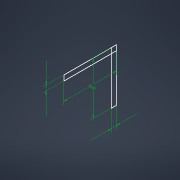
# Autodesk Inventor part: slide_panel_joint
Saved by Autodesk Inventor 2021 (Build 250183000, 183)
## iProperties
Created: 2023-03-31
Part Number: slide_panel_joint
Material: 一般
Document SubType Name: Modeling
Designer: casey
Density: 1 g/cm^3
Appearance: 既定
Author: casey
Autodesk Inventor part; units mm, degrees
ref_plane "YZ Plane" through (0, 0, 0) normal (1, 0, 0) x (0, 1, 0)
ref_plane "XZ Plane" through (0, 0, 0) normal (0, 1, 0) x (-1, 0, 0)
ref_plane "XY Plane" through (0, 0, 0) normal (0, 0, 1) x (1, 0, 0)
sketch "スケッチ1" plane through (0, 0, 0) normal (1, 0, 0) x (0, 1, 0)
  line L0 (0, 0) -> (-1, 0)
  line L1 (-1, 0) -> (-1, 10)
  line L2 (-1, 10) -> (0, 10)
  line L3 (0, 10) -> (0, 0)
  line L4 (0, 0) -> (-10, 0)
  line L5 (-10, 0) -> (-10, 1)
  line L6 (-10, 1) -> (0, 1)
  line L7 (0, 1) -> (0, 0)
  point P0 (-1, 1)
  dimension "d0" = 1
  dimension "d1" = 10
  dimension "d2" = 10
  dimension "d3" = 1
  constraints: 16 end point, 4 parallel, 2 horizontal, 2 perpendicular
  measures "d0" distance of L1.end L2.end
  measures "d1" distance of L0.end L1.end
  measures "d2" distance of L5.end L6.end
  measures "d3" distance of L4.end L5.end
extrude "押し出し1" add sketch "スケッチ1" along normal blind 130
sketch "スケッチ2" plane through (0, 0, 10) normal (0, 1, 0) x (1, 0, 0)
  line L0 (0, 10) -> (0, 0) projected
  line L1 (0, 10) -> (130, 10) projected
  line L2 (130, 10) -> (130, 0) projected
  point P0 (5, 5)
  point P1 (125, 5)
  dimension "d13" = 5
  dimension "d14" = 5
  dimension "d15" = 5
  dimension "d16" = 5
  measures "d13" distance from line of L0 point (5, 5)
  measures "d14" distance from line of L1 point (5, 5)
  measures "d15" distance from line of L2 point (125, 5)
  measures "d16" distance from line of point (125, 5) L1
hole "穴1" at (5, 0, 5) at (125, 0, 5) direction (0, -1, 0) diameter 3.5 end through all
sketch "スケッチ3" plane through (0, -10, 0) normal (0, 0, -1) x (-1, 0, 0)
  line L0 (0, 0) -> (-130, 0) projected
  line L1 (-130, 0) -> (-130, 10) projected
  line L2 (0, 0) -> (0, 10) projected
  point P0 (-115, 5)
  point P1 (-15, 5)
  dimension "d24" = 5
  dimension "d25" = 5
  dimension "d26" = 15
  dimension "d27" = 15
  measures "d24" distance from line of L0 point (-115, 5)
  measures "d25" distance from line of L0 point (-15, 5)
  measures "d26" distance from line of L1 point (-115, 5)
  measures "d27" distance from line of L2 point (-15, 5)
hole "穴2" at (115, -5, 0) at (15, -5, 0) direction (0, 0, 1) diameter 3.5 end through all
